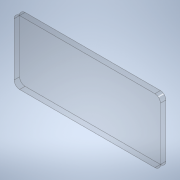
# Autodesk Inventor part: EW_Plexiglas
Saved by Autodesk Inventor 2020 (Build 240168000, 168)
## iProperties
Created: 2020-06-21
Part Number: EW_Plexiglas
Material: PMMA-Kunststoff
Document SubType Name: Modeling
Designer: Johannes
Density: 1.188 g/cm^3
Appearance: Rauchfarben - Schwarz
Author: Johannes
Autodesk Inventor part; units mm, degrees
ref_plane "YZ Plane" through (0, 0, 0) normal (1, 0, 0) x (0, 1, 0)
ref_plane "XZ Plane" through (0, 0, 0) normal (0, 1, 0) x (-1, 0, 0)
ref_plane "XY Plane" through (0, 0, 0) normal (0, 0, 1) x (1, 0, 0)
sketch "Skizze1" plane through (0, 0, 0) normal (0, 0, 1) x (1, 0, 0)
  line L0 (-40, 17.5) -> (40, 17.5)
  line L1 (40, 17.5) -> (40, -17.5)
  line L2 (40, -17.5) -> (-40, -17.5)
  line L3 (-40, -17.5) -> (-40, 17.5)
  line L4 (-40, 17.5) -> (40, -17.5) construction
  line L5 (40, 17.5) -> (-40, -17.5) construction
  point P0 (0, 0)
  dimension "d0" = 80
  dimension "d1" = 35
  constraints: 12 end point, 2 midpoint, 2 parallel, 1 horizontal, 1 perpendicular
  measures "d0" distance of L1.end L2.end
  measures "d1" distance of L0.end L1.end
extrude "Extrusion1" add sketch "Skizze1" along normal blind 3
fillet "Rundung1" radius 3 4 edges at (40, 17.5, 1.5) (40, -17.5, 1.5) (-40, -17.5, 1.5) (-40, 17.5, 1.5)
